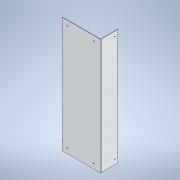
# Autodesk Inventor part: Laterales
Saved by Autodesk Inventor 2021 (Build 250183000, 183)
## iProperties
Created: 2021-04-18
Part Number: Laterales
Material: Acero ASTM A36
Document SubType Name: Chapa
Designer: carlo
Density: 7.85 g/cm^3
Sheet Metal Rule: Por defecto_mm
Appearance: Placa
Mass: 1750.88 g
Surface Area: 3740.72 cm^2
Volume: 223.042 cm^3
Flat Pattern Width: 31.3743 cm
Flat Pattern Length: 60 cm
Flat Pattern Area: 1882.46 cm^2
Sheet Metal Width: 313,743 mm
Sheet Metal Length: 600,000 mm
Sheet Metal Area: 188245,805 mm^2
Author: carlo
Autodesk Inventor part; units mm, degrees
ref_plane "YZ Plane" through (0, 0, 0) normal (1, 0, 0) x (0, 1, 0)
ref_plane "XZ Plane" through (0, 0, 0) normal (0, 1, 0) x (-1, 0, 0)
ref_plane "XY Plane" through (0, 0, 0) normal (0, 0, 1) x (1, 0, 0)
sketch "Boceto1" plane through (0, 0, 0) normal (0, 0, 1) x (1, 0, 0)
  line L0 (0, 0) -> (200, 0)
  line L1 (200, 0) -> (200, 600)
  line L2 (200, 600) -> (0, 600)
  line L3 (0, 600) -> (0, 0)
  dimension "d0" = 200
  dimension "d1" = 600
  measures "d0" distance of L2.end L1.end
  measures "d1" distance of L1.end L0.end
extrude "Placa1" add sketch "Boceto1" along normal blind 1.2
sketch "Boceto2" plane through (198.8, 600, 1.2) normal (1, 0, 0) x (0, 1, 0)
  line L0 (-600, 0) -> (0, 0)
  line L1 (0, 0) -> (0, 90)
  line L2 (0, 90) -> (-600, 90)
  line L3 (-600, 90) -> (-600, 0)
  constraints: 6 end point, 1 horizontal, 1 perpendicular, 1 vertical
edge flange "Pestaña1" height 90 angle -90 thickness 1.2 bend radius 1.2 thickness toward (1, 0, 0) relief straight relief width 1.2 relief depth 0.6 edges at (200, 300, 1.2) wall of the first edge with corners at (198.8, 0, 1.2) (198.8, 600, 1.2) (198.8, 600, -88.8) (198.8, 0, -88.8)
bend "Doblez1"
corner "Esquina1"
sketch "Boceto5" plane through (198.8, 0, -88.8) normal (0, 0, -1) x (-1, 0, 0)
  line L0 (-1.2, 600) -> (-1.2, 0)
  line L1 (-1.2, 47) -> (13.8, 47)
  line L2 (13.8, 47) -> (13.8, 553)
  line L3 (13.8, 553) -> (-1.2, 553)
  line L4 (-1.2, 553) -> (-1.2, 47)
  point P0 (198.8, 0)
  dimension "d17" = 15
  dimension "d18" = 506
  measures "d17" distance of L3.end L2.end
  measures "d18" distance of L2.end L1.end
sheet face with bend "Cara2" sketch "Boceto5" thickness 1.2 toward (0, 0, 1) bend radius 1.2 relief straight relief width 1.2 relief depth 0.6
bend "Doblez2"
sketch "Boceto6" plane through (0, 0, 0) normal (-1, 0, 0) x (0, 0, 1)
  line L0 (1.2, 0) -> (1.2, 600)
  line L1 (1.2, 47) -> (-13.8, 47)
  line L2 (-13.8, 47) -> (-13.8, 553)
  line L3 (-13.8, 553) -> (1.2, 553)
  line L4 (1.2, 553) -> (1.2, 47)
  point P0 (0, 0)
  dimension "d24" = 15
  dimension "d25" = 506
  measures "d24" distance of L2.end L3.end
  measures "d25" distance of L1.end L2.end
sheet face with bend "Cara3" sketch "Boceto6" thickness 1.2 toward (1, 0, 0) bend radius 1.2 relief straight relief width 1.2 relief depth 0.6
bend "Doblez3"
sketch "Boceto7" plane through (0, 0, 1.2) normal (0, 0, 1) x (1, 0, 0)
  circle A0 centre (164.262, 25) radius 2.5
  circle A1 centre (27.766, 25) radius 2.5
  line L0 (0, 47) -> (0, 553) projected
  line L1 (0, 300) -> (200, 300)
  line L2 (200, 47) -> (200, 553) projected
  circle A2 centre (164.262, 575) radius 2.5
  circle A3 centre (27.766, 575) radius 2.5
  line L3 (200, 600) -> (200, 0) projected
  line L4 (2.4, 47) -> (3, 47) projected
  line L5 (197.6, 0) -> (197.6, 600) projected
  line L6 (198.8, 0) -> (198.8, 600) projected
  point P0 (0, 0)
  dimension "d31" = 5
  dimension "d32" = 5
  dimension "d37" = 22
  dimension "d38" = 22
  dimension "d44" = 171.034
  dimension "d45" = 34.538
  constraints: 4 centre point, 2 end point, 2 midpoint, 2 symmetric about line, 2 other
  measures "d31" diameter of A0
  measures "d32" diameter of A1
  measures "d37" distance from line of A1.centre L4
  measures "d38" distance from line of A0.centre L4
  measures "d44" distance from line of A1.centre L6
  measures "d45" distance from line of L6 A0.centre
extrude "Extrusión1" cut sketch "Boceto7" against normal blind 5
sketch "Boceto8" plane through (200, 0, -1.2) normal (1, 0, 0) x (0, 0, -1)
  circle A0 centre (71.295, 575) radius 2.5
  line L0 (87.6, 47) -> (87.6, 553) projected
  line L1 (87.6, 300) -> (-2.4, 300)
  line L2 (-2.4, 0) -> (-2.4, 600) projected
  circle A1 centre (71.295, 25) radius 2.5
  line L3 (87.6, 554.2) -> (87.6, 600) projected
  line L4 (-1.2, 600) -> (-1.2, 0) projected
  line L5 (0, 600) -> (87.6, 600) projected
  dimension "d39" = 5
  dimension "d46" = 72.495
  dimension "d48" = 25
  constraints: 2 centre point, 2 end point, 2 midpoint, 1 symmetric about line, 1 other
  measures "d39" diameter of A0
  measures "d46" distance from line of A0.centre L4
  measures "d48" distance from line of L5 A0.centre
extrude "Extrusión2" cut sketch "Boceto8" against normal blind 5
thread "Thread1" size "M6x1" class "6H" standard "ISO Metric profile" full length
thread "Thread2" size "M6x1" class "6H" standard "ISO Metric profile" full length
thread "Thread3" size "M6x1" class "6H" standard "ISO Metric profile" full length
thread "Thread4" size "M6x1" class "6H" standard "ISO Metric profile" full length
thread "Thread5" size "M6x1" class "6H" standard "ISO Metric profile" full length
thread "Thread6" size "M6x1" class "6H" standard "ISO Metric profile" full length
equation "\"d2\" = Grosor"
equation "\"d3\" = Anchura_desahogo_plegado"
equation "\"d4\" = Profundidad_desahogo_plegado"
equation "\"d5\" = Remanente_mínimo"
equation "\"d6\" = Radiodetransición"
equation "\"d9\" = Radio_pliegue"
equation "\"d10\" = Tamaño_destalonado"
equation "\"d11\" = TamañoSeparación"
equation "\"d12\" = Tamaño_de_radio_de_Jacobi"
equation "\"d19\" = Radio_pliegue"
equation "\"d20\" = Anchura_desahogo_plegado"
equation "\"d22\" = Remanente_mínimo"
equation "\"d21\" = Profundidad_desahogo_plegado"
equation "\"d23\" = Radiodetransición"
equation "\"d26\" = Radio_pliegue"
equation "\"d27\" = Anchura_desahogo_plegado"
equation "\"d29\" = Remanente_mínimo"
equation "\"d28\" = Profundidad_desahogo_plegado"
equation "\"d30\" = Radiodetransición"
equation "\"Radio_pliegue\" = Grosor"
equation "\"Anchura_desahogo_plegado\" = Grosor"
equation "\"Radiodetransición\" = Radio_pliegue"
equation "\"Tamaño_de_radio_de_Jacobi\" = Radio_pliegue"
equation "\"TamañoSeparación\" = Grosor"
equation "\"Grosor\" = 1.2"
equation "\"Profundidad_desahogo_plegado\" = 0.6"
equation "\"Remanente_mínimo\" = 2.4"
equation "\"Tamaño_destalonado\" = 4.8"
